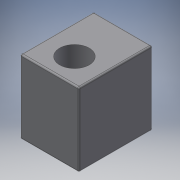
# Autodesk Inventor part: transmission box
Saved by Autodesk Inventor 2018 (Build 220112000, 112)
## iProperties
Created: 2017-12-24
Part Number: transmission box
Material: Generic
Document SubType Name: Modeling
Designer: Hembramone
Density: 1 g/cm^3
Appearance: Default
Author: Hembramone
Autodesk Inventor part; units mm, degrees
ref_plane "YZ Plane" through (0, 0, 0) normal (1, 0, 0) x (0, 1, 0)
ref_plane "XZ Plane" through (0, 0, 0) normal (0, 1, 0) x (-1, 0, 0)
ref_plane "XY Plane" through (0, 0, 0) normal (0, 0, 1) x (1, 0, 0)
sketch "Sketch1" plane through (0, 0, 0) normal (0, 0, 1) x (1, 0, 0)
  line L0 (4000, 5000) -> (4000, -5000)
  line L1 (4000, -5000) -> (-4000, -5000)
  line L2 (-4000, -5000) -> (-4000, 5000)
  line L3 (-4000, 5000) -> (4000, 5000)
  line L4 (4000, 5000) -> (-4000, -5000) construction
  line L5 (4000, -5000) -> (-4000, 5000) construction
  point P0 (0, 0)
  dimension "d0" = 10000
  dimension "d1" = 8000
  constraints: 12 end point, 2 midpoint, 2 parallel, 1 perpendicular, 1 vertical
  measures "d0" distance of L0.start L0.end
  measures "d1" distance of L0.end L1.end
extrude "Extrusion1" add sketch "Sketch1" along normal blind 10000
fillet "Fillet1" radius 200 12 edges at (4000, 0, 0) (0, -5000, 0) (4000, -5000, 5000) (4000, 5000, 5000) (0, 5000, 0) (-4000, 5000, 5000) (-4000, 0, 0) (-4000, -5000, 5000) (0, -5000, 10000) (-4000, 0, 10000) (4000, 0, 10000) (0, 5000, 10000)
sketch "Sketch2" plane through (0, 0, 0) normal (0, 0, -1) x (-1, 0, 0)
  circle A0 centre (0, 0) radius 1750 projected
  circle A1 centre (0, 0) radius 2250
  point P0 (0, 0)
  dimension "d5" = 4500
  constraints: 1 centre point, 1 coincident
  measures "d5" diameter of A1
extrude "Extrusion2" add sketch "Sketch2" along normal blind 1000
sketch "Sketch3" plane through (-3800, 5000, 9800) normal (0, 1, 0) x (1, 0, 0)
  circle A0 centre (3800, 3186.1125) radius 2000
  point P0 (3800, 9800)
  dimension "d8" = 4000
  constraints: 1 centre point
  measures "d8" diameter of A0
extrude "Extrusion3" cut sketch "Sketch3" against normal blind 4000
sketch "Sketch4" plane through (0, 1000, 6613.8875) normal (0, 1, 0) x (1, 0, 0)
  circle A0 centre (0, 0) radius 250
  point P0 (0, 6613.8875)
  dimension "d12" = 500
  constraints: 1 centre point
  measures "d12" diameter of A0
extrude "Extrusion4" cut sketch "Sketch4" against normal blind 4000
body "Solid1"
